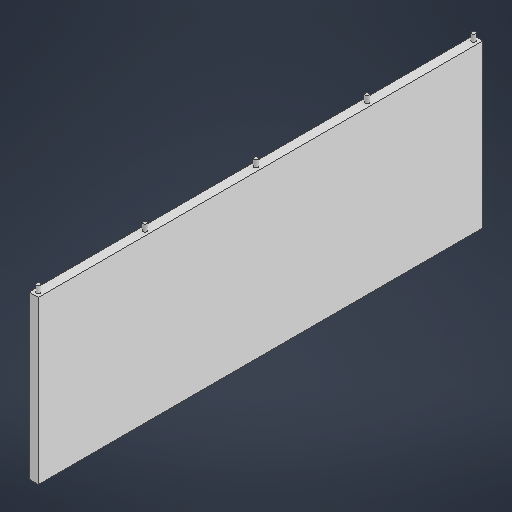
# Autodesk Inventor part: DindingKargoDepanBelakang
Saved by Autodesk Inventor 2026.1 (Build 301233020, 233B)
## iProperties
Created: 2025-11-09
Part Number: DindingKargoDepanBelakang
Material: Generic
Document SubType Name: Modeling
Designer: FrianVex
Density: 1 g/cm^3
Appearance: Default
Author: FrianVex
Autodesk Inventor part; units mm, degrees
ref_plane "YZ Plane" through (0, 0, 0) normal (1, 0, 0) x (0, 1, 0)
ref_plane "XZ Plane" through (0, 0, 0) normal (0, 1, 0) x (-1, 0, 0)
ref_plane "XY Plane" through (0, 0, 0) normal (0, 0, 1) x (1, 0, 0)
sketch "Sketch1" plane through (0, 0, 0) normal (0, 1, 0) x (-1, 0, 0)
  line L0 (2, -96) -> (-2, -96)
  line L1 (-2, -96) -> (-2, 96)
  line L2 (-2, 96) -> (2, 96)
  line L3 (2, 96) -> (2, -96)
  line L4 (2, -96) -> (-2, 96) construction
  line L5 (-2, -96) -> (2, 96) construction
  circle A0 centre (0, 94) radius 0.85
  circle A1 centre (0, -94) radius 0.85
  circle A2 centre (0, 0) radius 0.85
  circle A3 centre (0, 48) radius 0.85
  circle A4 centre (0, -48) radius 0.85
  point P0 (0, 0)
  dimension "d0" = 192
  dimension "d1" = 4
  dimension "d2" = 1.7
  dimension "d3" = 2
  dimension "d4" = 2
  dimension "d5" = 1.7
  dimension "d6" = 2
  dimension "d7" = 2
  dimension "d8" = 1.7
  dimension "d9" = 96
  dimension "d10" = 2
  dimension "d11" = 1.7
  dimension "d12" = 2
  dimension "d13" = 48
  dimension "d14" = 1.7
  dimension "d15" = 2
  dimension "d16" = 48
  constraints: 12 end point, 5 centre point, 2 midpoint, 2 parallel, 1 horizontal, 1 perpendicular
  measures "d0" distance of L0.end L1.end
  measures "d1" distance of L1.end L2.end
  measures "d2" diameter of A0
  measures "d3" distance from line of L2 A0.centre
  measures "d4" distance from line of L3 A0.centre
  measures "d5" diameter of A1
  measures "d6" distance from line of L3 A1.centre
  measures "d7" distance from line of L0 A1.centre
  measures "d8" diameter of A2
  measures "d9" distance from line of L2 A2.centre
  measures "d10" distance from line of L3 A2.centre
  measures "d11" diameter of A3
  measures "d12" distance from line of L3 A3.centre
  measures "d13" distance from line of L2 A3.centre
  measures "d14" diameter of A4
  measures "d15" distance from line of L3 A4.centre
  measures "d16" distance from line of L0 A4.centre
extrude "MainBody" add sketch "Sketch1" along normal blind 70
sketch "Sketch2" plane through (0, 70, 0) normal (0, 1, 0) x (1, 0, 0)
  circle A0 centre (0, 0) radius 0.85
  constraints: 1 centre point, 1 coincident
extrude "MiddlePole" add sketch "Sketch2" along normal blind 3 and the other way blind 70
sketch "Sketch3" plane through (0, 70, 0) normal (0, 1, 0) x (1, 0, 0)
  circle A0 centre (0, -48) radius 0.85
  point P0 (0, 0)
  constraints: 1 centre point
extrude "MiddleLeftPole" add sketch "Sketch3" along normal blind 3 and the other way blind 70
sketch "Sketch4" plane through (0, 70, 0) normal (0, 1, 0) x (1, 0, 0)
  circle A0 centre (0, -94) radius 0.85
  point P0 (0, 0)
  constraints: 1 centre point
extrude "LeftMostPole" add sketch "Sketch4" along normal blind 3 and the other way blind 70
sketch "Sketch5" plane through (0, 70, 0) normal (0, 1, 0) x (1, 0, 0)
  circle A0 centre (0, 48) radius 0.85
  point P0 (0, 0)
  constraints: 1 centre point
extrude "Extrusion5" add sketch "Sketch5" along normal blind 3 and the other way blind 70
sketch "Sketch6" plane through (0, 70, 0) normal (0, 1, 0) x (1, 0, 0)
  circle A0 centre (0, 94) radius 0.85
  point P0 (0, 0)
  constraints: 1 centre point
extrude "Extrusion6" add sketch "Sketch6" along normal blind 3 and the other way blind 70
body "Solid1"
